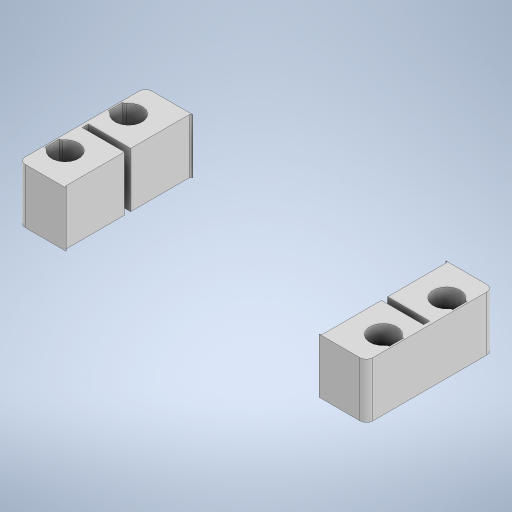
# Autodesk Inventor part: buh2
Saved by Autodesk Inventor 2024 (Build 280153000, 153)
## iProperties
Created: 2024-02-07
Part Number: buh2
Material: Generic
Document SubType Name: Modeling
Designer: jebes windows
Density: 1 g/cm^3
Appearance: Default
Author: jebes windows
## iProperties of the stored document buh2_3DPrint.ipt
Created: 2024-02-07
Part Number: buh2_3DPrint
Material: Generic
Document SubType Name: Modeling
Designer: jebes windows
Density: 1 g/cm^3
Appearance: Default
Author: jebes windows
Autodesk Inventor part; units mm, degrees
ref_plane "YZ Plane" through (0, 0, 0) normal (1, 0, 0) x (0, 1, 0)
ref_plane "XZ Plane" through (0, 0, 0) normal (0, 1, 0) x (-1, 0, 0)
ref_plane "XY Plane" through (0, 0, 0) normal (0, 0, 1) x (1, 0, 0)
ref_plane "Work Plane1" through (25.1605, -6.525, -8.5) normal (0, 0, 1) x (1, 0, 0)
sketch "Sketch2" plane through (25.1605, -6.525, -8.5) normal (0, 0, 1) x (1, 0, 0)
  line L0 (-6.8105, 7) -> (-6.8105, 16.075) projected
  line L1 (-6.8105, 7) -> (-0.2605, 7) projected
  line L2 (-0.2605, 7) -> (-0.2605, 6.05) projected
  line L3 (-6.8105, 6.05) -> (-0.2605, 6.05) projected
  line L4 (-6.8105, -3.025) -> (-6.8105, 6.05) projected
  arc A0 (-7.1105, -3.325) -> (-6.8105, -3.025) centre (-7.1105, -3.025) ccw projected
  line L5 (-7.1105, -3.325) -> (-0.7605, -3.325) projected
  arc A1 (-0.7605, -3.325) -> (0.2395, -2.325) centre (-0.7605, -2.325) ccw projected
  line L6 (0.2395, -2.325) -> (0.2395, 0.5) projected
  line L7 (0.2395, 0.5) -> (0, 0.5) projected
  arc A2 (0, 0.5) -> (-0.3941, 0.3077) centre (0, 0) ccw projected
  arc A3 (-0.3941, 2.8923) -> (-0.3941, 0.3077) centre (-2.0494, 1.6) ccw projected
  arc A4 (-0.3941, 2.8923) -> (0, 2.7) centre (0, 3.2) ccw projected
  line L8 (0, 2.7) -> (0.2395, 2.7) projected
  line L9 (0.2395, 2.7) -> (0.2395, 10.35) projected
  line L10 (0.2395, 10.35) -> (0, 10.35) projected
  arc A5 (0, 10.35) -> (-0.3941, 10.1577) centre (0, 9.85) ccw projected
  arc A6 (-0.3941, 12.7423) -> (-0.3941, 10.1577) centre (-2.0494, 11.45) ccw projected
  arc A7 (-0.3941, 12.7423) -> (0, 12.55) centre (0, 13.05) ccw projected
  line L11 (0, 12.55) -> (0.2395, 12.55) projected
  line L12 (0.2395, 12.55) -> (0.2395, 15.375) projected
  arc A8 (0.2395, 15.375) -> (-0.7605, 16.375) centre (-0.7605, 15.375) ccw projected
  line L13 (-0.7605, 16.375) -> (-7.1105, 16.375) projected
  arc A9 (-6.8105, 16.075) -> (-7.1105, 16.375) centre (-7.1105, 16.075) ccw projected
  line L14 (-53.2605, 7) -> (-53.2605, 6.05) projected
  line L15 (-46.7105, 7) -> (-53.2605, 7) projected
  line L16 (-46.7105, 16.075) -> (-46.7105, 7) projected
  arc A10 (-46.4105, 16.375) -> (-46.7105, 16.075) centre (-46.4105, 16.075) ccw projected
  line L17 (-46.4105, 16.375) -> (-52.7605, 16.375) projected
  arc A11 (-52.7605, 16.375) -> (-53.7605, 15.375) centre (-52.7605, 15.375) ccw projected
  line L18 (-53.7605, 15.375) -> (-53.7605, 12.55) projected
  line L19 (-53.7605, 12.55) -> (-53.5211, 12.55) projected
  arc A12 (-53.5211, 12.55) -> (-53.127, 12.7423) centre (-53.5211, 13.05) ccw projected
  arc A13 (-53.127, 10.1577) -> (-53.127, 12.7423) centre (-51.4717, 11.45) ccw projected
  arc A14 (-53.127, 10.1577) -> (-53.5211, 10.35) centre (-53.5211, 9.85) ccw projected
  line L20 (-53.5211, 10.35) -> (-53.7605, 10.35) projected
  line L21 (-53.7605, 10.35) -> (-53.7605, 2.7) projected
  line L22 (-53.7605, 2.7) -> (-53.5211, 2.7) projected
  arc A15 (-53.5211, 2.7) -> (-53.127, 2.8923) centre (-53.5211, 3.2) ccw projected
  arc A16 (-53.127, 0.3077) -> (-53.127, 2.8923) centre (-51.4717, 1.6) ccw projected
  arc A17 (-53.127, 0.3077) -> (-53.5211, 0.5) centre (-53.5211, 0) ccw projected
  line L23 (-53.5211, 0.5) -> (-53.7605, 0.5) projected
  line L24 (-53.7605, 0.5) -> (-53.7605, -2.325) projected
  arc A18 (-53.7605, -2.325) -> (-52.7605, -3.325) centre (-52.7605, -2.325) ccw projected
  line L25 (-52.7605, -3.325) -> (-46.4105, -3.325) projected
  arc A19 (-46.7105, -3.025) -> (-46.4105, -3.325) centre (-46.4105, -3.025) ccw projected
  line L26 (-46.7105, 6.05) -> (-46.7105, -3.025) projected
  line L27 (-46.7105, 6.05) -> (-53.2605, 6.05) projected
  line L28 (-53.5211, 0.5) -> (-53.5211, 2.7)
  line L29 (-53.7605, 0.5) -> (-53.7605, 2.7)
  line L30 (-53.7605, 10.35) -> (-53.7605, 12.55)
  line L31 (-53.5211, 10.35) -> (-53.5211, 12.55)
  line L32 (0.2395, 0.5) -> (0.2395, 2.7)
  line L33 (0, 0.5) -> (0, 2.7)
  line L34 (0.2395, 10.35) -> (0.2395, 12.55)
  line L35 (0, 10.35) -> (0, 12.55)
  point P0 (-25.1605, 6.525)
  constraints: 16 end point, 7 vertical, 1 collinear
ref_plane "Work Plane2" through (-11.5498, -16.6818, 0) normal (0, 0, 1) x (1, 0, 0)
extrude "Extrusion1" add sketch "Sketch2" along normal up to surface (8.5 mm away) contours L0 A9 L13 A8 L12 L11 A7 A6 A5 L10 L9 L8 A4 A3 A2 L7 L6 A1 L5 A0 L4 L3 L2 L1 | L34 L10 L35 L11 | L32 L7 L33 L8 | L14 L27 L26 A19 L25 A18 L24 L23 A17 A16 A15 L22 L21 L20 A14 A13 A12 L19 L18 A11 L17 A10 L16 L15 | L19 L31 L20 L30 | L29 L22 L28 L23
body "Solid1"
